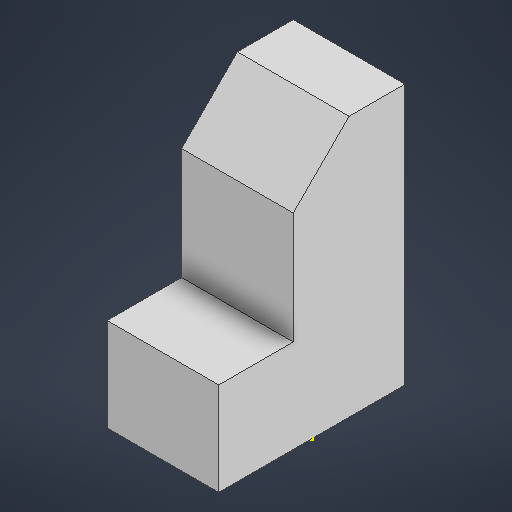
# Autodesk Inventor part: Peça1
Saved by Autodesk Inventor 2027.1 (Build 311270010, 270A)
## iProperties
Created: 2026-09-24
Part Number: Peça1
Material: Genérico
Document SubType Name: Modeling
Designer: carlo
Density: 1 g/cm^3
Appearance: Padrão
Author: carlo
Autodesk Inventor part; units mm, degrees
ref_plane "YZ Plane" through (0, 0, 0) normal (1, 0, 0) x (0, 1, 0)
ref_plane "XZ Plane" through (0, 0, 0) normal (0, 1, 0) x (-1, 0, 0)
ref_plane "XY Plane" through (0, 0, 0) normal (0, 0, 1) x (1, 0, 0)
sketch "Esboço1" plane through (0, 0, 0) normal (0, 1, 0) x (-1, 0, 0)
  line L0 (-15, 25) -> (15, 25)
  line L1 (15, 25) -> (15, -25)
  line L2 (15, -25) -> (-15, -25)
  line L3 (-15, -25) -> (-15, 25)
  line L4 (-15, 25) -> (15, -25) construction
  line L5 (15, 25) -> (-15, -25) construction
  point P0 (0, 0)
  dimension "d0" = 30
  dimension "d1" = 50
  constraints: 12 end point, 2 midpoint, 2 parallel, 1 horizontal, 1 perpendicular
  measures "d0" distance of L1.end L2.end
  measures "d1" distance of L0.end L1.end
extrude "Extrusão1" add sketch "Esboço1" along normal blind 70
sketch "Esboço2" plane through (15, 0, 25) normal (1, 0, 0) x (0, 0, -1)
  point P0 (25, 0)
sketch "Esboço3" plane through (15, 0, 25) normal (1, 0, 0) x (0, 0, -1)
  point P0 (25, 0)
sketch "Esboço4" plane through (15, 0, 25) normal (1, 0, 0) x (0, 0, -1)
  line L0 (0, 70) -> (20, 70)
  line L1 (20, 70) -> (20, 25)
  line L2 (20, 25) -> (0, 25)
  line L3 (0, 25) -> (0, 70)
  line L4 (50, 0) -> (50, 70) projected
  line L5 (0, 0) -> (50, 0) projected
  point P0 (25, 0)
  dimension "d4" = 30
  dimension "d5" = 25
  constraints: 8 end point, 2 parallel, 1 coincident, 1 horizontal, 1 perpendicular
  measures "d4" distance between parallel lines of L1 L4
  measures "d5" distance between parallel lines of L2 L5
extrude "Extrusão2" cut sketch "Esboço4" against normal blind 30
sketch "Esboço5" plane through (15, 0, 25) normal (1, 0, 0) x (0, 0, -1)
  point P0 (25, 0)
chamfer "Chanfro1" distance 15 angle 45 1 edges at (0, 70, 5) measured on face at (5, 70, -5)
